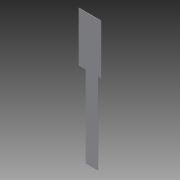
# Autodesk Inventor part: La
Saved by Autodesk Inventor 2014 SP1 (Build 180222100, 222)
## iProperties
Created: 2015-03-28
Part Number: La
Material: LCP Plastic
Document SubType Name: Modeling
Designer: tuleu
Density: 1.626 g/cm^3
Appearance: PVC - White
Author: tuleu
Autodesk Inventor part; units mm, degrees
ref_plane "YZ Plane" through (0, 0, 0) normal (1, 0, 0) x (0, 1, 0)
ref_plane "XZ Plane" through (0, 0, 0) normal (0, 1, 0) x (-1, 0, 0)
ref_plane "XY Plane" through (0, 0, 0) normal (0, 0, 1) x (1, 0, 0)
sketch "Sketch1" plane through (0, 0, 0) normal (0, 1, 0) x (-1, 0, 0)
  line L0 (35, -525) -> (-65, -525)
  line L1 (-90, 125) -> (-90, 525)
  line L2 (-90, 525) -> (90, 525)
  line L3 (-65, -525) -> (-65, 125)
  line L4 (-65, 125) -> (-90, 125)
  line L5 (0, 525) -> (0, -525)
  line L6 (35, -525) -> (35, 125)
  line L7 (35, 125) -> (90, 125)
  line L8 (90, 525) -> (90, 125)
  line L9 (35, 0) -> (-65, 0)
  point P0 (0, 0)
  dimension "d2" = 650
  dimension "d6" = 1050
  dimension "d7" = 180
  dimension "d8" = 55
  dimension "d9" = 155
  constraints: 20 end point, 5 perpendicular, 4 parallel, 4 point on line, 2 midpoint, 1 collinear, 1 horizontal, 1 other
  measures "d2" distance of L0.end L3.end
  measures "d6" distance between parallel lines of L2 L0
  measures "d7" distance of L1.end L2.end
  measures "d8" distance between parallel lines of L6 L8
  measures "d9" distance between parallel lines of L3 L8
extrude "Extrusion1" add sketch "Sketch1" along normal blind 2
body "Solid1"
